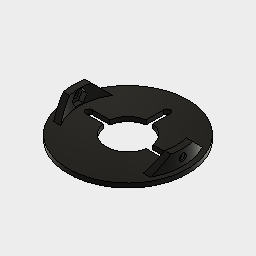
Camera Tube Mount (Autodesk Fusion 360 design; units mm, degrees)
Autodesk Fusion 360 part; units mm, degrees
sketch "Sketch1" plane through (0, 0, 0) normal (0, 1, 0) x (1, 0, 0)
  circle A0 centre (0, 0) radius 27.5
  circle A1 centre (0, 0) radius 10
  line L0 (0, 0) -> (13, 0)
  line L1 (0, 0) -> (0, 13)
  line L2 (0, 0) -> (-13, 0)
  line L3 (-13, 0) -> (-13, 1.55)
  line L4 (-13, 1.55) -> (-18, 1.55)
  line L5 (-13, 1.55) -> (-9.8791, 1.55)
  line L6 (-13, 0) -> (-13, -1.55)
  line L7 (-13, -1.55) -> (-9.8791, -1.55)
  line L8 (-13, -1.55) -> (-18, -1.55)
  line L9 (0, 13) -> (1.55, 13)
  line L10 (1.55, 13) -> (1.55, 18)
  line L11 (1.55, 18) -> (-1.55, 18)
  line L12 (-1.55, 18) -> (-1.55, 9.8791)
  line L13 (1.55, 9.8791) -> (1.55, 18)
  line L14 (13, 0) -> (13, -1.55)
  line L15 (13, -1.55) -> (18, -1.55)
  line L16 (18, -1.55) -> (9.8791, -1.55)
  line L17 (9.8791, 1.55) -> (18, 1.55)
  line L18 (18, 1.55) -> (18, -1.55)
  arc A2 (-18, 1.55) -> (-18, -1.55) centre (-18, 0) ccw
  arc A3 (1.55, 18) -> (-1.55, 18) centre (0, 18) ccw
  arc A4 (18, -1.55) -> (18, 1.55) centre (18, 0) ccw
  dimension "d12" = 13
  dimension "d13" = 13
  dimension "d14" = 13
  dimension "d15" = 1.55
  dimension "d16" = 5
  dimension "d17" = 1.55
  dimension "d18" = 1.55
  dimension "d19" = 5
  dimension "d20" = 3.1
  dimension "d21" = 1.55
  dimension "d22" = 5
  dimension "d23" = 3.1
  measures "d12" distance of A0.centre L0.end
  measures "d13" distance of A0.centre L1.end
  measures "d14" distance of A0.centre L2.end
  measures "d15" distance of L2.end L3.end
  measures "d16" distance of L3.end L4.end
  measures "d17" distance of L2.end L6.end
  measures "d18" distance of L1.end L9.end
  measures "d19" distance of L9.end L10.end
  measures "d20" distance of L10.end L11.end
  measures "d21" distance of L0.end L14.end
  measures "d22" distance of L14.end L15.end
  measures "d23" distance of L15.end L17.end
extrude "Extrude1" add sketch "Sketch1" along normal blind 2
sketch "Sketch2" plane through (0, 2, 0) normal (0, 1, 0) x (-1, 0, 0)
  line L0 (-18, 1.55) -> (-9.8791, 1.55)
  arc A0 (9.8791, 1.55) -> (-9.8791, 1.55) centre (0, 0) ccw
  line L1 (9.8791, 1.55) -> (18, 1.55)
  arc A1 (18, -1.55) -> (18, 1.55) centre (18, 0) ccw
  line L2 (18, -1.55) -> (9.8791, -1.55)
  arc A2 (1.55, -9.8791) -> (9.8791, -1.55) centre (0, 0) ccw
  line L3 (1.55, -9.8791) -> (1.55, -18)
  arc A3 (-1.55, -18) -> (1.55, -18) centre (0, -18) ccw
  line L4 (-1.55, -18) -> (-1.55, -9.8791)
  arc A4 (-9.8791, -1.55) -> (-1.55, -9.8791) centre (0, 0) ccw
  line L5 (-9.8791, -1.55) -> (-18, -1.55)
  arc A5 (-18, 1.55) -> (-18, -1.55) centre (-18, 0) ccw
  circle A6 centre (0, 0) radius 27.5
  circle A7 centre (0, 0) radius 25.3
  circle A8 centre (0, 0) radius 22.5
  dimension "d26" = 50.6
  dimension "d27" = 45
  measures "d26" diameter of A7
  measures "d27" diameter of A8
extrude "Extrude2" add sketch "Sketch2" along normal blind 7 contours A7
ref_plane "WorkPlane2" through (25.5, 0, 0) normal (1, 0, 0) x (0, 1, 0)
sketch "Sketch4" plane through (25.5, 0, 0) normal (1, 0, 0) x (0, 0, -1)
  line L0 (0, 9) -> (0, 5.5)
  circle A0 centre (0, 5.5) radius 1.6
  point P0 (0, 9)
  dimension "d35" = 3.5
  dimension "d36" = 3.2
  measures "d35" distance of P0 L0.end
  measures "d36" diameter of A0
extrude "Extrude4" cut sketch "Sketch4" against normal through all
ref_plane "WorkPlane3" through (22.5, 0, 0) normal (1, 0, 0) x (0, 1, 0)
sketch "Sketch5" plane through (22.5, 0, 0) normal (1, 0, 0) x (0, 0, -1)
  line L0 (-1.7321, 8.5) -> (-3.4641, 5.5)
  line L1 (-3.4641, 5.5) -> (-1.7321, 2.5)
  line L2 (-1.7321, 2.5) -> (1.7321, 2.5)
  line L3 (1.7321, 2.5) -> (3.4641, 5.5)
  line L4 (3.4641, 5.5) -> (1.7321, 8.5)
  line L5 (1.7321, 8.5) -> (-1.7321, 8.5)
  point P0 (0, 5.5)
extrude "Extrude5" cut sketch "Sketch5" along normal blind 2 and the other way blind 1
pattern_circular "C-Pattern1" count 2 over 360 about axis through (0, 1.75, 0) along (0, 1, 0) of "Extrude5"
sketch "Sketch6" plane through (0, 0, 0) normal (1, 0, 0) x (0, 0, -1)
  line L0 (0, 9) -> (-2, 9)
  line L1 (1.55, 2) -> (9.8791, 2)
  line L2 (27.5, 2) -> (-27.5, 2)
  line L3 (28, 9) -> (28, 2)
  line L4 (28, 2) -> (-25.7716, 2)
  line L5 (-25.7716, 2) -> (-25.7716, 9)
  line L6 (0, 9) -> (-5, 9)
  line L7 (0, 9) -> (5, 9)
  line L8 (5, 9) -> (12, 2)
  line L9 (5, 9) -> (14.8995, 9) construction
  line L10 (-5, 9) -> (-12, 2)
  line L11 (28, 9) -> (-26, 9)
  point P0 (0, 9)
  dimension "d46" = 2
  dimension "d52" = 5
  dimension "d53" = 5
  dimension "d54" = 45
  measures "d46" distance of P0 L0.end
  measures "d52" distance of P0 L6.end
  measures "d53" distance of P0 L7.end
  measures "d54" angle of L8 L9
extrude "Extrude8" cut sketch "Sketch6" along normal mid plane 57.44 contours L2 L3 L4 L8 L11 | L2 L4 L5 L10 L11
